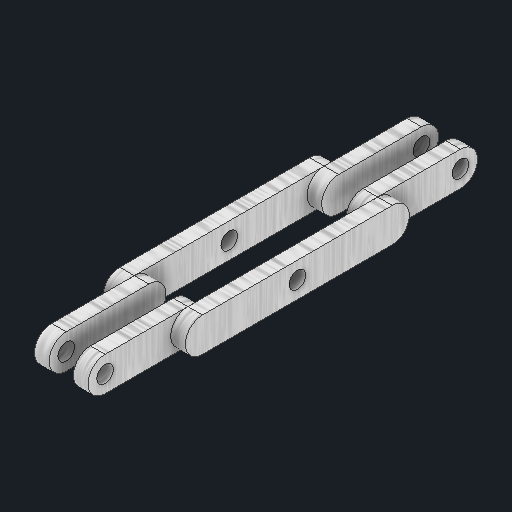
# Autodesk Inventor part: Corredera I
Saved by Autodesk Inventor 2025.3 (Build 293356030, 356C)
## iProperties
Created: 2024-11-12
Part Number: Corredera I
Material: Aluminum 7075
Document SubType Name: Modeling
Designer: j.santaa
Density: 2.81 g/cm^3
Appearance: Satin - Brushed Heavy
Author: j.santaa
Autodesk Inventor part; units mm, degrees
ref_plane "YZ Plane" through (0, 0, 0) normal (1, 0, 0) x (0, 1, 0)
ref_plane "XZ Plane" through (0, 0, 0) normal (0, 1, 0) x (-1, 0, 0)
ref_plane "XY Plane" through (0, 0, 0) normal (0, 0, 1) x (1, 0, 0)
sketch "Sketch1" plane through (0, 0, 0) normal (1, 0, 0) x (0, 1, 0)
  line L0 (0, -36.5) -> (0, 36.5) construction
  line L1 (3.5, -36.5) -> (3.5, 36.5)
  line L2 (-3.5, 36.5) -> (-3.5, -36.5)
  arc A0 (-3.5, -36.5) -> (3.5, -36.5) centre (0, -36.5) ccw
  arc A1 (3.5, 36.5) -> (-3.5, 36.5) centre (0, 36.5) ccw
  circle A2 centre (0, 36.5) radius 1.5
  circle A3 centre (0, -36.5) radius 1.5
  line L3 (0, -19.5) -> (0, 19.5) construction
  line L4 (3.5, -19.5) -> (3.5, 19.5)
  line L5 (-3.5, 19.5) -> (-3.5, -19.5)
  arc A4 (-3.5, -19.5) -> (3.5, -19.5) centre (0, -19.5) ccw
  arc A5 (3.5, 19.5) -> (-3.5, 19.5) centre (0, 19.5) ccw
  line L6 (0, -36.5) -> (0, -19.5) construction
  line L7 (-3.5, -36.5) -> (-3.5, -19.5)
  line L8 (3.5, -19.5) -> (3.5, -36.5)
  arc A6 (-3.5, -36.5) -> (3.5, -36.5) centre (0, -36.5) ccw
  arc A7 (3.5, -19.5) -> (-3.5, -19.5) centre (0, -19.5) ccw
  line L9 (3.5, 0) -> (-3.5, 0) construction
  line L10 (0, 36.5) -> (0, 19.5) construction
  line L11 (-3.5, 36.5) -> (-3.5, 19.5)
  line L12 (3.5, 19.5) -> (3.5, 36.5)
  arc A8 (3.5, 36.5) -> (-3.5, 36.5) centre (0, 36.5) ccw
  arc A9 (-3.5, 19.5) -> (3.5, 19.5) centre (0, 19.5) ccw
  circle A10 centre (0, 0) radius 1.5
  point P0 (0, 0)
  point P1 (0, -40)
  point P2 (0, 40)
  point P3 (3.5, 19.5)
  point P4 (-3.5, 19.5)
  point P5 (3.5, -19.5)
  point P6 (0, -28)
  point P7 (0, 28)
  point P8 (3.5, 19.5)
  point P9 (-3.5, 19.5)
  point P10 (-3.5, -19.5)
  point P11 (3.5, -19.5)
  point P12 (0, 0)
  point P13 (0, 0)
  dimension "d18" = 80
  dimension "d20" = 7
  dimension "d32" = 39
  dimension "d44" = 3
  dimension "d46" = 0
  constraints: 34 end point, 18 point on circle, 16 tangent, 11 centre point, 8 midpoint, 5 equal radius, 4 parallel, 3 coincident, 2 collinear, 1 point on line, 1 symmetric about line, 1 vertical
  measures "d18" distance of point (0, -40) point (0, 40)
  measures "d20" diameter of A1
  measures "d32" distance of L3.start L3.end
  measures "d44" diameter of A10
  measures "d46" distance of point (0, 0) A10.centre
extrude "Extrusión3" add sketch "Sketch1" along normal mid plane 17 contours A7 L2 A9 L1 | A4 A7 | A9 A5 | A10
extrude "Extrusión4" cut sketch "Sketch1" along normal mid plane 11 contours A7 L2 A9 L1 | A4 A7 | A9 A5 | A10
extrude "Extrusión5" add sketch "Sketch1" along normal mid plane 11 contours A0 L2 A4 L1 | A4 A7 | A5 L2 A1 L1 | A9 A5 | A2 | A3
extrude "Extrusión6" cut sketch "Sketch1" along normal mid plane 5 contours A0 L2 A4 L1 | A4 A7 | A5 L2 A1 L1 | A9 A5 | A2 | A3
sketch "Boceto2" plane through (-5.5, 0, 0) normal (-1, 0, 0) x (0, 0, 1)
  point P0 (-36.5, 0)
  point P1 (36.5, 0)
hole "Agujero1" at (-5.5, 0, -36.5) at (-5.5, 0, 36.5) direction (1, 0, 0) diameter 3.4 end through all clearance for "Tornillo de cabeza plana avellanada ISO 2009/7046" size "M3" standard "ISO"
sketch "Boceto3" plane through (8.5, 0, 0) normal (1, 0, 0) x (0, 0, -1)
  point P0 (0, 0)
  point P1 (0, 0)
hole "Agujero2" at (8.5, 0, 0) direction (-1, 0, 0) diameter 3.4 end through all clearance for "Tornillo de cabeza plana avellanada ISO 2009/7046" size "M3" standard "ISO"
